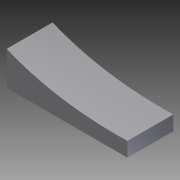
# Autodesk Inventor part: ruber1
Saved by Autodesk Inventor 2012 (Build 160160000, 160)
## iProperties
Created: 2013-08-22
Part Number: ruber1
Material: Default
Document SubType Name: Modeling
Designer: Dantro
Density: 1 g/cm^3
Author: Dantro
Autodesk Inventor part; units mm, degrees
ref_plane "YZ Plane" through (0, 0, 0) normal (1, 0, 0) x (0, 1, 0)
ref_plane "XZ Plane" through (0, 0, 0) normal (0, 1, 0) x (-1, 0, 0)
ref_plane "XY Plane" through (0, 0, 0) normal (0, 0, 1) x (1, 0, 0)
sketch "Sketch1" plane through (0, 0, 0) normal (0, 0, 1) x (1, 0, 0)
  line L0 (0, 0) -> (25, 0)
  line L1 (25, 0) -> (25, 3)
  line L2 (0, 7) -> (0, 0)
  spline S0 degree 2 poles (0, 7) (10.4974, 2.6328) (25, 3) knots 0 0 0 1 1 1
  line L3 (22.1754, 2.9285) -> (27.8246, 3.0715) construction
  arc A0 (22.7403, 2.9709) -> (27.2583, 3.0853) centre (22.6995, 93.8518) ccw construction
  point P0 (10.7252, 3.9454)
  dimension "d1" = 25
  dimension "d2" = 7
  dimension "d5" = 3
  constraints: 8 end point, 2 midpoint, 1 centre point, 1 horizontal, 1 parallel, 1 perpendicular, 1 point on circle, 5 other
  measures "d1" distance of L0.start L0.end
  measures "d2" distance of L0.start L2.start
  measures "d5" distance of L0.end L1.end
extrude "Extrusion1" add sketch "Sketch1" along normal blind 9.5
body "Solid1"
